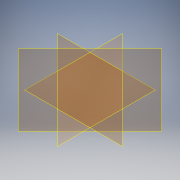
# Autodesk Inventor part: Foot thing
Saved by Autodesk Inventor 2019 (Build 230136000, 136)
## iProperties
Created: 2022-04-03
Part Number: Foot thing
Material: Generic
Document SubType Name: Modeling
Designer: Ian
Density: 1 g/cm^3
Appearance: Default
Author: Ian
Autodesk Inventor part; units mm, degrees
ref_plane "XZ Plane" through (0, 0, 0) normal (0, 1, 0) x (-1, 0, 0)
ref_plane "Work Plane1" through (0, 0, 0) normal (0.7071, 0, 0.7071) x (0, -1, 0)
sketch "Sketch1" plane through (0, 0, 0) normal (0.7071, 0, 0.7071) x (0, -1, 0)
  line L0 (-9, 0) -> (-9, 10)
  line L1 (-9, 10) -> (-4, 10)
  line L2 (-4, 10) -> (-4, 0)
  line L3 (-4, 0) -> (0, 0)
  line L4 (0, 0) -> (0, 13)
  line L5 (0, 13) -> (49, 73)
  line L6 (49, 73) -> (49, 82.7959)
  line L7 (49, 82.7959) -> (44, 82.7959)
  line L8 (44, 82.7959) -> (-13, 13)
  line L9 (-13, 13) -> (-13, 0)
  line L10 (-13, 0) -> (-9, 0)
  line L11 (0, -16.5592) -> (0, 99.3551) projected
  line L12 (0, 0) -> (-5.3698, 0) construction
  dimension "d0" = 4
  dimension "d1" = 4
  dimension "d2" = 5
  dimension "d3" = 10
  dimension "d4" = 3
  dimension "d5" = 60
  dimension "d6" = 5
  dimension "d8" = 53
  constraints: 24 end point, 6 perpendicular, 3 parallel, 2 point on line, 1 collinear, 1 horizontal, 1 horizontal alignment, 1 vertical
  measures "d0" distance of L9.end L0.start
  measures "d1" distance of L2.end L3.end
  measures "d2" distance of L0.end L1.end
  measures "d3" distance of L0.start L0.end
  measures "d4" vertical distance of L0.end L8.end
  measures "d5" vertical distance of L4.end L5.end
  measures "d6" distance of L6.end L7.end
  measures "d8" distance between parallel lines of L6 L2
extrude "Extrusion1" add sketch "Sketch1" along normal blind 10
sketch "Sketch2" plane through (0, 13, 0) normal (0, 1, 0) x (0.7071, 0, 0.7071)
  circle A0 centre (5, 5) radius 2.55
  line L0 (0, 0) -> (0, 10) projected
  line L1 (0, 5) -> (5, 0)
  line L2 (0, 0) -> (10, 0) projected
  line L3 (5, 0) -> (10, 5)
  line L4 (10, 13) -> (10, 0) projected
  line L5 (2.5, 2.5) -> (5, 5) construction
  line L6 (5, 5) -> (7.5, 2.5) construction
  dimension "d11" = 5.1
  dimension "d12" = 45
  dimension "d13" = 45
  constraints: 8 end point, 4 midpoint, 3 perpendicular, 1 centre point, 1 point on line
  measures "d11" diameter of A0
  measures "d12" angle of L0 L1
  measures "d13" angle of L4 L3
extrude "Extrusion2" cut sketch "Sketch2" against normal through all
fillet "Fillet1" radius 2 2 edges at (3.5355, 2, 3.5355) (3.5355, 11, 3.5355)
body "Solid1"
